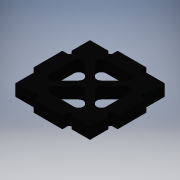
# Autodesk Inventor part: 上腕_メインフレーム_1_1
Saved by Autodesk Inventor 2018 (Build 220112000, 112)
## iProperties
Created: 2016-05-04
Part Number: 上腕_メインフレーム_1_1
Material: アセタール樹脂、黒
Document SubType Name: Modeling
Designer: hiroaki
Density: 1.425 g/cm^3
Appearance: 滑らか - 黒
Mass: 5.46708 g
Surface Area: 31.8962 cm^2
Volume: 3.83655 cm^3
d0: 32.500 mm
d1: 1.050 mm
d2: 2.000 mm
d3: 10.000 mm
d4: 3.100 mm
d6: 3.000 mm
d8: 3.000 mm
d9: 3.000 mm
d10: 3.000 mm
d11: 3.000 mm
d12: 3.000 mm
d13: 4.000 mm
d14: 2.500 mm
d15: 0.00 deg
d17: 5.000 mm
d18: 5.000 mm
d30: 2.000 mm
Author: hiroaki
Autodesk Inventor part; units mm, degrees
ref_plane "YZ Plane" through (0, 0, 0) normal (1, 0, 0) x (0, 1, 0)
ref_plane "XZ Plane" through (0, 0, 0) normal (0, 1, 0) x (-1, 0, 0)
ref_plane "XY Plane" through (0, 0, 0) normal (0, 0, 1) x (1, 0, 0)
sketch "スケッチ1" plane through (0, 0, 0) normal (0, 0, 1) x (1, 0, 0)
  line L0 (-16.25, -16.25) -> (16.25, -16.25) construction
  line L1 (16.25, -16.25) -> (16.25, 16.25) construction
  line L2 (16.25, 16.25) -> (-16.25, 16.25) construction
  line L3 (-16.25, 16.25) -> (-16.25, -16.25) construction
  line L4 (-16.25, -16.25) -> (16.25, 16.25) construction
  line L5 (16.25, -16.25) -> (-16.25, 16.25) construction
  line L6 (-8.35, 16.25) -> (-16.25, 16.25)
  line L7 (-16.25, 16.25) -> (-16.25, 8.35)
  line L8 (8.35, 16.25) -> (16.25, 16.25)
  line L9 (16.25, 16.25) -> (16.25, 8.35)
  line L10 (-16.25, -8.35) -> (-16.25, -16.25)
  line L11 (-16.25, -16.25) -> (-8.35, -16.25)
  line L12 (8.35, -16.25) -> (16.25, -16.25)
  line L13 (16.25, -16.25) -> (16.25, -8.35)
  line L14 (-6.25, 16.25) -> (-6.25, 18.25)
  line L15 (-6.25, 18.25) -> (6.25, 18.25)
  line L16 (6.25, 18.25) -> (6.25, 16.25)
  arc A0 (-8.35, 16.25) -> (-6.25, 16.25) centre (-7.3, 16.25) ccw
  arc A1 (6.25, 16.25) -> (8.35, 16.25) centre (7.3, 16.25) ccw
  line L17 (0, 16.25) -> (0, 0) construction
  line L18 (0, 0) -> (16.25, 0) construction
  line L19 (-16.25, 6.25) -> (-18.25, 6.25)
  line L20 (-18.25, 6.25) -> (-18.25, -6.25)
  line L21 (-18.25, -6.25) -> (-16.25, -6.25)
  arc A2 (-16.25, 6.25) -> (-16.25, 8.35) centre (-16.25, 7.3) ccw
  arc A3 (-16.25, -8.35) -> (-16.25, -6.25) centre (-16.25, -7.3) ccw
  line L22 (-6.25, -16.25) -> (-6.25, -18.25)
  line L23 (-6.25, -18.25) -> (6.25, -18.25)
  line L24 (6.25, -18.25) -> (6.25, -16.25)
  arc A4 (-6.25, -16.25) -> (-8.35, -16.25) centre (-7.3, -16.25) ccw
  arc A5 (8.35, -16.25) -> (6.25, -16.25) centre (7.3, -16.25) ccw
  line L25 (16.25, 6.25) -> (18.25, 6.25)
  line L26 (18.25, 6.25) -> (18.25, -6.25)
  line L27 (18.25, -6.25) -> (16.25, -6.25)
  arc A6 (16.25, 8.35) -> (16.25, 6.25) centre (16.25, 7.3) ccw
  arc A7 (16.25, -6.25) -> (16.25, -8.35) centre (16.25, -7.3) ccw
  line L28 (-12.8, 16.25) -> (-9.7, 16.25) construction
  line L29 (-9.7, 16.25) -> (-9.7, 13.25) construction
  line L30 (-9.7, 13.25) -> (-12.8, 13.25) construction
  line L31 (-12.8, 13.25) -> (-12.8, 16.25) construction
  line L32 (-16.25, 12.8) -> (-13.25, 12.8) construction
  line L33 (-13.25, 12.8) -> (-13.25, 9.7) construction
  line L34 (-13.25, 9.7) -> (-16.25, 9.7) construction
  line L35 (-16.25, 9.7) -> (-16.25, 12.8) construction
  line L36 (-10.1287, 12.25) -> (10.1287, 12.25)
  line L37 (10.1287, 12.25) -> (0, 2.1213)
  line L38 (0, 2.1213) -> (-10.1287, 12.25)
  line L39 (-12.25, 10.1287) -> (-12.25, -10.1287)
  line L40 (-12.25, -10.1287) -> (-2.1213, 0)
  line L41 (-2.1213, 0) -> (-12.25, 10.1287)
  line L42 (-10.1287, -12.25) -> (10.1287, -12.25)
  line L43 (10.1287, -12.25) -> (0, -2.1213)
  line L44 (0, -2.1213) -> (-10.1287, -12.25)
  line L45 (12.25, 10.1287) -> (12.25, -10.1287)
  line L46 (12.25, -10.1287) -> (2.1213, 0)
  line L47 (2.1213, 0) -> (12.25, 10.1287)
  line L48 (-11.25, 16.25) -> (-11.25, 13.25) construction
  line L49 (-13.25, 11.25) -> (-16.25, 11.25) construction
  dimension "d0" = 32.5
  dimension "d1" = 1.05
  dimension "d2" = 2
  dimension "d3" = 10
  dimension "d4" = 3.1
  dimension "d6" = 3
  dimension "d8" = 3
  dimension "d9" = 3
  dimension "d10" = 3
  dimension "d11" = 3
  dimension "d12" = 3
  dimension "d13" = 4
  dimension "d17" = 5
  dimension "d18" = 5
  constraints: 100 end point, 17 perpendicular, 16 point on circle, 13 parallel, 9 horizontal, 8 centre point, 8 midpoint, 8 tangent, 7 equal length, 7 equal radius, 6 symmetric about line, 5 collinear, 5 vertical, 4 horizontal alignment, 4 vertical alignment, 10 other
  measures "d0" distance of L2.end L0.start
  measures "d1" radius of A0
  measures "d2" distance between parallel lines of L2 L15
  measures "d3" distance between parallel lines of L3 L14
  measures "d4" distance of L28.start L28.end
  measures "d6" distance between parallel lines of L6 L30
  measures "d8" distance between parallel lines of L3 L33
  measures "d9" distance between parallel lines of L43 L46
  measures "d10" distance between parallel lines of L41 L38
  measures "d11" distance between parallel lines of L47 L37
  measures "d12" distance between parallel lines of L44 L40
  measures "d13" distance between parallel lines of L36 L2
  measures "d17" distance between parallel lines of L2 L49
  measures "d18" distance between parallel lines of L7 L48
extrude "押し出し1" add sketch "スケッチ1" along normal blind 2.5
mirror "ミラー1" about plane through (0, 0, 0) normal (0, 0, -1) of "押し出し1"
fillet "フィレット1" radius 2 12 edges at (12.25, 10.1287, 0) (12.25, -10.1287, 0) (10.1287, -12.25, 0) (0, 2.1213, 0) (-2.1213, 0, 0) (-10.1287, -12.25, 0) (-12.25, -10.1287, 0) (10.1287, 12.25, 0) (-12.25, 10.1287, 0) (-10.1287, 12.25, 0) (0, -2.1213, 0) (2.1213, 0, 0)
equation "\"d8\" = d6"
equation "\"d10\" = d9"
equation "\"d11\" = d10"
equation "\"d12\" = d11"
equation "\"d18\" = d17"
